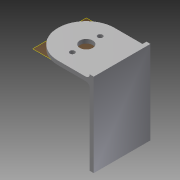
# Autodesk Inventor part: console
Saved by Autodesk Inventor 2015 SP1 (Build 190203100, 203)
## iProperties
Created: 2015-03-20
Part Number: console
Material: Ogólny
Document SubType Name: Modeling
Designer: Marcin
Density: 1 g/cm^3
Appearance: Stal
Author: Marcin
Autodesk Inventor part; units mm, degrees
ref_plane "YZ Plane" through (0, 0, 0) normal (1, 0, 0) x (0, 1, 0)
ref_plane "XZ Plane" through (0, 0, 0) normal (0, 1, 0) x (-1, 0, 0)
ref_plane "XY Plane" through (0, 0, 0) normal (0, 0, 1) x (1, 0, 0)
ref_plane "Płaszczyzna konstrukcyjna1" through (0, 0, 0) normal (0, 0, 1) x (1, 0, 0)
sketch "Szkic1" plane through (0, 0, 0) normal (0, 0, 1) x (1, 0, 0)
  circle A0 centre (0, 0) radius 12.25 projected
  circle A1 centre (0, 7) radius 1.2295 projected
  circle A2 centre (0, -7) radius 1.2295 projected
  circle A3 centre (0, 0) radius 17.25
  line L0 (0, -17.25) -> (16, -17.25)
  line L1 (16, -17.25) -> (16, 17.25)
  line L2 (16, 17.25) -> (0, 17.25)
  line L3 (0, 17.25) -> (0, -17.25)
  point P0 (0, 0)
  dimension "d0" = 5
  dimension "d1" = 16
  constraints: 8 end point, 2 parallel, 2 tangent, 1 centre point, 1 horizontal, 1 midpoint, 1 perpendicular
  measures "d0" radial gap between concentric circles of A0 A3
  measures "d1" distance from line of point (0, 0) L1
extrude "Wyciągnięcie proste1" add sketch "Szkic1" along normal blind 2
sketch "Szkic2" plane through (0, 0, 2) normal (0, 0, 1) x (1, 0, 0)
  arc A0 (-1.3229, 1.5) -> (1.3229, 1.5) centre (0, 0) ccw projected
  circle A1 centre (0, 7) radius 1.2295 projected
  circle A2 centre (0, -7) radius 1.2295 projected
  circle A3 centre (0, 0) radius 3.25 projected
  point P0 (0, 0)
extrude "Wyciągnięcie proste2" cut sketch "Szkic2" against normal up to next
sketch "Szkic3" plane through (16, -17.25, 0) normal (1, 0, 0) x (0, 0, -1)
  line L0 (0, 0) -> (0, 10.8031) projected
  line L1 (0, 34.5) -> (-2, 34.5) projected
  line L2 (-2, 0) -> (-2, 10.8031) projected
  line L3 (0, 0) -> (-2, 0) projected
  line L4 (-2, 34.5) -> (-2, 34.5)
  line L5 (-2, 34.5) -> (-2, 0)
  line L6 (-2, 0) -> (-2, 0)
  line L7 (-2, 0) -> (-2, 34.5)
  line L8 (0, 0) -> (-2, 0) projected
  line L9 (-2, 34.5) -> (-2, 34.5)
  line L10 (-2, 34.5) -> (-2, 0)
  line L11 (-2, 0) -> (-2, 0)
  line L12 (-2, 0) -> (-2, 34.5)
  line L13 (0, 10.8031) -> (-2, 10.8031) projected
  line L14 (-2, 23.6969) -> (0, 23.6969) projected
  line L15 (0, 23.6969) -> (0, 34.5) projected
  line L16 (-2, 23.6969) -> (-2, 34.5) projected
  point P0 (0, 17.25)
  dimension "d6" = 0
  dimension "d9" = 0
  constraints: 16 end point, 4 collinear, 2 horizontal, 2 parallel, 2 perpendicular, 1 midpoint, 1 point on line
  measures "d6" distance of L1.end L4.end
  measures "d9" distance of L10.end L11.end
extrude "Wyciągnięcie proste3" add sketch "Szkic3" along normal blind 2
sketch "Szkic5" plane through (0, 0, 2) normal (0, 0, 1) x (1, 0, 0)
  line L0 (0, 17.25) -> (18, 17.25) projected
  line L1 (0, -17.25) -> (18, -17.25) projected
  line L2 (0, -17.25) -> (18, -17.25) projected
  line L3 (18, 17.25) -> (9, 17.25)
  line L4 (9, 17.25) -> (9, -17.25)
  line L5 (9, -17.25) -> (18, -17.25)
  line L6 (18, -17.25) -> (18, 17.25)
  point P0 (0, 0)
  constraints: 8 end point, 2 parallel, 1 horizontal, 1 midpoint, 1 perpendicular
extrude "Wyciągnięcie proste4" add sketch "Szkic5" against normal up to surface (2 mm away)
ref_plane "Płaszczyzna konstrukcyjna2" through (0, 12.25, 2) normal (0, 1, 0) x (1, 0, 0)
sketch "Szkic7" plane through (0, 12.25, 2) normal (0, 1, 0) x (1, 0, 0)
  line L0 (0, 0) -> (18, 0) projected
  line L1 (18, 0) -> (18, -18)
  line L2 (18, -18) -> (0, 0)
  point P0 (0, 2)
  constraints: 4 end point, 1 perpendicular, 1 vertical
extrude "Wyciągnięcie proste6" add sketch "Szkic7" along normal mid plane 2
mirror "Odbicie lustrzane1" about plane through (0, 0, 0) normal (0, 1, 0) of "Wyciągnięcie proste6"
ref_plane "Płaszczyzna konstrukcyjna3" through (0, 0, 0) normal (0, 1, 0) x (-1, 0, 0)
